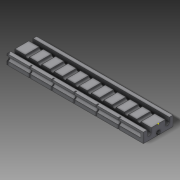
# Autodesk Inventor part: Track Builder
Saved by Autodesk Inventor 2015 SP1 (Build 190203100, 203)
## iProperties
Created: 2015-05-13
Part Number: Track Builder
Material: Generic
Document SubType Name: Modeling
Designer: Andrew
Density: 1 g/cm^3
Appearance: Default
Author: Andrew
Autodesk Inventor part; units mm, degrees
ref_plane "YZ Plane" through (0, 0, 0) normal (1, 0, 0) x (0, 1, 0)
ref_plane "XZ Plane" through (0, 0, 0) normal (0, 1, 0) x (-1, 0, 0)
ref_plane "XY Plane" through (0, 0, 0) normal (0, 0, 1) x (1, 0, 0)
sketch "Sketch1" plane through (0, 0, 0) normal (0, 0, 1) x (1, 0, 0)
  circle A0 centre (0, 0) radius 8.6875 construction
  arc A1 (-8.9597, -7.3097) -> (-5.6597, -7.3097) centre (-7.3097, -7.3097) ccw
  circle A2 centre (7.3097, -7.3097) radius 1.65 construction
  line L0 (0, 12.8169) -> (0, -16.0892) projected
  line L1 (-7.3097, -8.9597) -> (7.3097, -8.9597) construction
  line L2 (0, 0) -> (7.3097, -7.3097) construction
  line L3 (11.9597, -4.0097) -> (11.9597, -11.9597)
  line L4 (11.9597, -11.9597) -> (-11.9597, -11.9597)
  line L5 (-11.9597, -11.9597) -> (-11.9597, -4.0097)
  circle A3 centre (-7.3097, -4.0097) radius 1.65 construction
  line L6 (-8.9597, -7.3097) -> (-8.9597, -4.0097)
  line L7 (-5.6597, -7.3097) -> (-5.6597, -4.0097)
  line L8 (-11.9597, -4.0097) -> (-8.9597, -4.0097)
  arc A4 (5.6597, -7.3097) -> (8.9597, -7.3097) centre (7.3097, -7.3097) ccw
  line L9 (8.9597, -7.3097) -> (8.9597, -4.0097)
  line L10 (5.6597, -7.3097) -> (5.6597, -4.0097)
  line L11 (-5.6597, -4.0097) -> (5.6597, -4.0097)
  line L12 (8.9597, -4.0097) -> (11.9597, -4.0097)
  dimension "d0" = 17.375
  dimension "d1" = 3.3
  dimension "d4" = 45
  dimension "d5" = 3
  dimension "d6" = 4.65
  dimension "d25" = 17.9194
  constraints: 24 end point, 7 point on circle, 6 tangent, 4 centre point, 4 horizontal, 4 parallel, 4 symmetric about line, 3 perpendicular, 2 equal radius, 2 vertical alignment, 1 coincident, 5 other
  measures "d0" diameter of A0
  measures "d1" diameter of A1
  measures "d4" angle of L0 L2
  measures "d5" distance between parallel lines of L5 L6
  measures "d6" distance from line of L4 A1.centre
  measures "d25" distance between parallel lines of L6 L9
extrude "Extrusion1" add sketch "Sketch1" along normal blind 110
sketch "Sketch2" plane through (5.6597, -7.3097, 0) normal (1, 0, 0) x (0, 0, -1)
  line L0 (0, -4.65) -> (0, 3.3) projected
  line L1 (0, 3.3) -> (-110, 3.3) projected
  line L2 (-110, -4.65) -> (-110, 3.3) projected
  line L3 (0, -4.65) -> (-110, -4.65) projected
  line L4 (0, 3.3) -> (-110, 3.3) projected
  circle A0 centre (-10, 3.3) radius 1.65
  point P0 (0, 7.3097)
  dimension "d9" = 10
  dimension "d10" = 3.3
  constraints: 1 centre point, 1 point on line
  measures "d9" distance from line of L0 A0.centre
  measures "d10" diameter of A0
extrude "Extrusion2" cut sketch "Sketch2" against normal up to surface (11.3194 mm away) contours A0 L1 | L1 A0
pattern_linear "Rectangular Pattern1" count 10 spacing 10 along (0, 0, 1) of "Extrusion2"
sketch "Sketch3" plane through (0, 0, 0) normal (0, 0, -1) x (-1, 0, 0)
  line L0 (11.9597, -4.0097) -> (11.9597, -11.9597) projected
  line L1 (8.9597, -4.0097) -> (11.9597, -4.0097) projected
  line L2 (8.9597, -7.3097) -> (8.9597, -4.0097) projected
  arc A0 (5.6597, -7.3097) -> (8.9597, -7.3097) centre (7.3097, -7.3097) ccw projected
  line L3 (5.6597, -4.0097) -> (5.6597, -7.3097) projected
  line L4 (-5.6597, -4.0097) -> (5.6597, -4.0097) projected
  line L5 (-5.6597, -7.3097) -> (-5.6597, -4.0097) projected
  arc A1 (-8.9597, -7.3097) -> (-5.6597, -7.3097) centre (-7.3097, -7.3097) ccw projected
  line L6 (-8.9597, -4.0097) -> (-8.9597, -7.3097) projected
  line L7 (-11.9597, -4.0097) -> (-8.9597, -4.0097) projected
  line L8 (-11.9597, -11.9597) -> (-11.9597, -4.0097) projected
  line L9 (11.9597, -11.9597) -> (-11.9597, -11.9597) projected
  arc A2 (0.375, -11.5665) -> (-0.375, -11.5665) centre (0, -9.9597) ccw
  line L10 (-0.375, -11.5665) -> (-0.375, -11.9597)
  line L11 (0.375, -11.5665) -> (0.375, -11.9597)
  point P0 (0, 0)
  dimension "d16" = 3.3
  dimension "d17" = 0.75
  dimension "d20" = 2
  constraints: 4 end point, 2 perpendicular, 2 point on circle, 2 point on line, 1 centre point, 1 parallel, 1 vertical alignment
  measures "d16" diameter of A2
  measures "d17" distance between parallel lines of L10 L11
  measures "d20" distance from line of L9 A2.centre
extrude "Extrusion3" cut sketch "Sketch3" against normal blind 30 contours L9 L10 A2 L11
sketch "Sketch4" plane through (-11.9597, -11.9597, 110) normal (0, -1, 0) x (1, 0, 0)
  line L0 (12.3347, -80) -> (12.3347, -110) projected
  line L1 (12.3347, -110) -> (23.9194, -110) projected
  line L2 (23.9194, -110) -> (23.9194, 0) projected
  line L3 (0, 0) -> (23.9194, 0) projected
  line L4 (0, -110) -> (0, 0) projected
  line L5 (0, -110) -> (11.5847, -110) projected
  line L6 (11.5847, -110) -> (11.5847, -80) projected
  line L7 (11.5847, -80) -> (12.3347, -80) projected
  line L8 (13.6097, -80) -> (10.3097, -80)
  line L9 (10.3097, -80) -> (10.3097, -83)
  line L10 (10.3097, -83) -> (13.6097, -83)
  line L11 (13.6097, -83) -> (13.6097, -80)
  line L12 (11.9597, 22) -> (11.9597, -132) projected
  point P0 (11.9597, -110)
  dimension "d21" = 3.3
  dimension "d22" = 3
  constraints: 8 end point, 2 collinear, 2 parallel, 1 horizontal, 1 perpendicular, 1 other
  measures "d21" distance between parallel lines of L11 L9
  measures "d22" distance between parallel lines of L8 L10
extrude "Extrusion4" cut sketch "Sketch4" against normal blind 2 contours L8 L11 L10 L0 | L0 L10 L12 L7 | L12 L10 L6 L7 | L6 L10 L9 L8
sketch "Sketch5" plane through (0, 0, 0) normal (0, 0, -1) x (-1, 0, 0)
  line L0 (-11.9597, -11.9597) -> (-11.9597, -4.0097) projected
  circle A0 centre (-11.9597, -7.3097) radius 1.65
  line L1 (-0.375, -11.9597) -> (-11.9597, -11.9597) projected
  line L2 (-11.9597, -4.0097) -> (-8.9597, -4.0097) projected
  point P0 (0, 0)
  dimension "d26" = 3.3
  dimension "d28" = 3.3
  constraints: 1 centre point, 1 point on line
  measures "d26" diameter of A0
  measures "d28" distance from line of L2 A0.centre
extrude "Extrusion5" cut sketch "Sketch5" against normal up to surface (110 mm away)
sketch "Sketch6" plane through (11.9597, -11.9597, 110) normal (1, 0, 0) x (0, 0, -1)
  line L0 (110, 0) -> (0, 0) projected
  line L1 (110, 7.95) -> (0, 7.95) projected
  line L2 (90.4556, 0) -> (89.7056, 0)
  line L3 (89.7056, 0) -> (89.7056, 7.95)
  line L4 (89.7056, 7.95) -> (90.4556, 7.95)
  line L5 (90.4556, 7.95) -> (90.4556, 0)
  line L6 (110, 0) -> (0, 0) construction
  line L7 (90.0806, 0) -> (90.0806, 7.95) construction
  line L8 (110, 7.95) -> (110, 4.65) projected
  line L9 (110, 3) -> (0, 3) projected
  line L10 (110, 6.3) -> (108, 6.3)
  line L11 (108, 6.3) -> (108, 3)
  line L12 (108, 3) -> (110, 3)
  line L13 (110, 3) -> (110, 6.3)
  point P0 (110, 11.9597)
  dimension "d31" = 0.75
  dimension "d32" = 2
  dimension "d33" = 17.9194
  constraints: 18 end point, 4 parallel, 4 point on line, 2 horizontal, 2 midpoint, 2 perpendicular
  measures "d31" distance between parallel lines of L3 L5
  measures "d32" distance of L10.start L10.end
  measures "d33" distance between parallel lines of L11 L7
extrude "Extrusion6" add sketch "Sketch6" against normal blind 1.65 contours L11 L10 L8 L13 L9
extrude "Extrusion7" cut sketch "Sketch6" against normal blind 1.65 contours L0 L3 L9 L5 | L9 L3 L1 L5
pattern_linear "Rectangular Pattern2" count 10 spacing 17.9194 along (0, 0, 1) of "Extrusion7"
sketch "Sketch7" plane through (-5.6597, -4.0097, 11.65) normal (0, 1, 0) x (1, 0, 0)
  point P0 (5.6597, 11.65)
equation "\"d0\" = marbleSize"
equation "\"d1\" = trackDiameter"
equation "\"d10\" = trackDiameter"
equation "\"d16\" = trackDiameter"
equation "\"d21\" = trackDiameter"
equation "\"d26\" = trackDiameter"
equation "\"d28\" = trackDiameter"
equation "\"d29\" = 0.5 * trackDiameter"
equation "\"d33\" = d25"
equation "\"d34\" = 0.5 * trackDiameter"
equation "\"d36\" = 0.5 * trackDiameter"
equation "\"d40\" = d25"
equation "\"marbleSize\" = 17.375"
equation "\"trackDiameter\" = 3.3"
body "Solid1"
